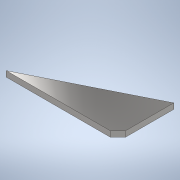
# Autodesk Inventor part: 21015-22-1-2- Floor Plate Gussets
Saved by Autodesk Inventor 2022 (Build 260153000, 153)
## iProperties
Created: 2021-06-17
Part Number: 21015-22-1-2- Floor Plate Gussets
Material: Steel, Carbon
Document SubType Name: Modeling
Designer: Skynet
Density: 7.85 g/cm^3
Appearance: Semi-Polished
Mass: 678.367 g
Surface Area: 228.956 cm^2
Volume: 86.4162 cm^3
Author: Skynet
Autodesk Inventor part; units mm, degrees
ref_plane "YZ Plane" through (0, 0, 0) normal (1, 0, 0) x (0, 1, 0)
ref_plane "XZ Plane" through (0, 0, 0) normal (0, 1, 0) x (-1, 0, 0)
ref_plane "XY Plane" through (0, 0, 0) normal (0, 0, 1) x (1, 0, 0)
sketch "Sketch1" plane through (0, 0, 0) normal (0, 1, 0) x (-1, 0, 0)
  line L0 (12.7, 0) -> (190.5, 0)
  line L1 (190.5, 0) -> (0, -95.25)
  line L2 (0, -95.25) -> (0, -12.7)
  line L3 (12.7, 0) -> (0, -12.7)
  point P0 (0, 0)
  dimension "d0" = 190.5
  dimension "d1" = 95.25
  dimension "d4" = 12.7
  dimension "d5" = 12.7
  constraints: 8 end point, 1 horizontal, 1 perpendicular
  measures "d0" distance of point (0, 0) L0.end
  measures "d1" distance of L1.end point (0, 0)
  measures "d4" distance of L0.start point (0, 0)
  measures "d5" distance of L2.end point (0, 0)
extrude "Extrusion1" add sketch "Sketch1" along normal blind 9.525
body "Solid1"
